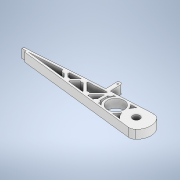
# Autodesk Inventor part: airfoil
Saved by Autodesk Inventor 2022 (Build 260153000, 153)
## iProperties
Created: 2021-03-06
Part Number: airfoil
Material: ABS Plastic
Document SubType Name: Modeling
Designer: Ferdinand Hubbard
Density: 1.06 g/cm^3
Appearance: Smooth - White
Mass: 36.0694 g
Surface Area: 132.212 cm^2
Volume: 34.0278 cm^3
Author: Ferdinand Hubbard
Autodesk Inventor part; units mm, degrees
ref_plane "YZ Plane" through (0, 0, 0) normal (1, 0, 0) x (0, 1, 0)
ref_plane "XZ Plane" through (0, 0, 0) normal (0, 1, 0) x (-1, 0, 0)
ref_plane "XY Plane" through (0, 0, 0) normal (0, 0, 1) x (1, 0, 0)
sketch "Sketch1" plane through (0, 0, 0) normal (0, 1, 0) x (-1, 0, 0)
  circle A0 centre (258.2631, 4.8308) radius 8
  spline S0 degree 4 poles (33.6209, 29.2007) (29.9061, 27.8418) (22.7215, 24.7905) (13.1918, 19.0698) (6.0464, 12.5974) (2.8487, 8.0358) (1.9781, 6.5052) knots 0 0 0 0 0 0.454638 0.631605 1 1 1 1 1
  line L0 (228.9693, 19.6719) -> (363.9561, 4.4165)
  circle A1 centre (370.8368, 3.6389) radius 4 construction
  circle A2 centre (234.1104, 5.3693) radius 11.5
  circle A3 centre (234.1104, 5.3693) radius 4
  circle A4 centre (206.3773, 7.0182) radius 8
  spline S1 degree 4 poles (6.5181, -5.2335) (7.1495, -5.5884) (14.4655, -7.5139) (22.7138, -8.7119) (35.9318, -9.9587) (48.9048, -10.4891) (62.2875, -10.9022) (78.073, -11.0572) (94.7047, -11.0677) (112.5814, -10.9208) (131.2146, -10.6471) (157.3003, -10.1275) (178.3649, -9.5608) (196.5129, -9.0389) (204.4707, -8.6918) knots 0 0 0 0 0 0.111052 0.17228 0.238392 0.309085 0.383789 0.461593 0.542487 0.625611 0.710417 0.796372 1 1 1 1 1
  line L1 (205.2712, 22.3501) -> (205.101, 22.3693)
  arc A5 (366.8619, 4.0863) -> (366.7774, 4.0976) centre (366.5513, 2.0974) ccw
  arc A6 (211.7482, -3.4099) -> (211.7084, 17.1634) centre (183.2631, 6.8218) ccw
  arc A7 (222.579, 17.5321) -> (220.8357, -4.8625) centre (234.1104, 5.3693) ccw
  arc A8 (211.7084, 17.1634) -> (205.101, 22.3693) centre (204.2043, 14.4352) ccw
  arc A9 (228.9693, 19.6719) -> (222.579, 17.5321) centre (228.0726, 11.7377) ccw
  arc A10 (204.4851, -8.6914) -> (211.7482, -3.4099) centre (204.2336, -0.7107) ccw
  arc A11 (220.8357, -4.8625) -> (227.4114, -7.9687) centre (227.1598, 0.0119) ccw
  line L2 (205.101, 22.3693) -> (228.9693, 19.6719)
  line L3 (204.4851, -8.6914) -> (227.4114, -7.9687)
  circle A12 centre (13.7692, 4.0714) radius 9.5
  circle A13 centre (13.7692, 4.0714) radius 8
  line L4 (6.5182, 10.2092) -> (6.4686, 10.2473)
  line L5 (6.5182, -2.0664) -> (6.4884, -2.0928)
  line L6 (6.3757, -3.4734) -> (8.2772, -5.8071)
  line L7 (6.2474, 11.5971) -> (7.6235, 13.6492)
  line L8 (7.6237, 9.1932) -> (7.4155, 9.361)
  line L9 (7.1111, 10.503) -> (8.7725, 14.7639)
  line L10 (7.7078, -1.1496) -> (7.6551, -1.1925)
  line L11 (7.6239, -2.4062) -> (12.536, -6.8462)
  arc A14 (6.4884, -2.0928) -> (6.3757, -3.4734) centre (7.151, -2.8417) ccw
  arc A15 (7.6551, -1.1925) -> (7.6239, -2.4062) centre (8.1604, -1.8127) ccw
  arc A16 (7.1111, 10.503) -> (7.4155, 9.361) centre (8.0428, 10.1397) ccw
  arc A17 (6.2474, 11.5971) -> (6.4686, 10.2473) centre (7.078, 11.0402) ccw
  circle A18 centre (206.3773, 7.0182) radius 9.5
  circle A19 centre (258.2631, 4.8308) radius 9.5
  line L12 (199.715, 25.2636) -> (204.715, 25.2636)
  line L13 (204.715, 21.8532) -> (204.715, 20.2636)
  line L14 (204.715, 20.2636) -> (199.715, 20.2636)
  line L15 (199.715, 20.2636) -> (199.715, 22.0923)
  line L16 (363.9561, 7.3621) -> (368.9561, 7.3621)
  line L17 (368.9561, 7.3621) -> (368.9561, 2.3621)
  line L18 (368.9561, 2.3621) -> (363.9561, 2.3621)
  line L19 (363.9561, 2.3621) -> (363.9561, 7.3621)
  line L20 (368.9561, 2.3621) -> (368.9561, 1.9548)
  arc A20 (367.0002, -0.0447) -> (368.9561, 1.9548) centre (366.9561, 1.9548) ccw
  spline S2 degree 4 poles (227.4114, -7.9687) (227.4417, -8.4597) (246.8106, -6.9409) (262.2854, -6.6719) (283.9243, -5.4893) (299.9375, -4.6081) (314.7418, -3.6091) (328.1615, -2.6489) (339.8305, -1.7709) (352.2883, -0.8813) (359.936, -0.3777) (366.0141, -0.1162) (366.8685, -0.083) knots 0 0 0 0 0 0.205018 0.312148 0.416329 0.516516 0.612219 0.702513 0.786392 0.862444 1 1 1 1 1
  spline S3 degree 4 poles (369.983, -0.0016) (369.9988, -0.0007) (370.0055, 0.0002) (370.0019, 0.001) (369.9872, 0.0018) knots 0 0 0 0 0 1 1 1 1 1
  line L21 (369.9445, -0.0037) -> (370.0215, 0.0006) construction
  arc A21 (369.9522, -0.0026) -> (370.0137, 0.0008) centre (369.9433, 0.7095) ccw construction
  line L22 (367.0002, -0.0447) -> (366.8685, -0.083)
  line L23 (34.5887, 29.5265) -> (39.5887, 29.5265)
  line L24 (39.5887, 26.3775) -> (39.5887, 24.5265)
  line L25 (39.5887, 24.5265) -> (34.5887, 24.5265)
  line L26 (34.5887, 24.5265) -> (34.5887, 28.83)
  line L27 (199.2285, 22.5921) -> (40.1023, 26.8773)
  arc A22 (16.4456, -7.6263) -> (9.2191, 15.1753) centre (13.7692, 4.0714) ccw
  spline S4 degree 3 poles (32.0186, 25.4505) (29.3529, 24.7737) (18.93, 19.4324) (14.8642, 16.0213) knots 0 0 0 0 1 1 1 1
  line L28 (39.5871, 22.0265) -> (34.5871, 22.0023)
  line L29 (32.0186, 25.4505) -> (32.0186, 21.9899)
  line L30 (32.0186, 21.9899) -> (34.5871, 22.0023)
  line L31 (39.5871, 22.0265) -> (42.0871, 22.0265)
  line L32 (42.0871, 24.1952) -> (42.0871, 22.0265)
  line L33 (197.2217, 20.4462) -> (197.2167, 17.9462)
  line L34 (197.2167, 17.9462) -> (207.215, 17.7637)
  line L35 (42.0871, 24.1952) -> (197.2217, 20.4462)
  line L36 (207.215, 17.7637) -> (207.215, 20.2046)
  line L37 (207.215, 20.2046) -> (361.1854, 2.2896)
  line L38 (361.1854, 2.2896) -> (361.2414, 2.3344)
  spline S5 degree 4 poles (21.2323, -5.3255) (22.7398, -5.5867) (33.0484, -6.8576) (45.6907, -7.3689) (62.672, -7.914) (78.3439, -8.0583) (95.0315, -8.0733) (112.8578, -7.9245) (131.5947, -7.6509) (162.8597, -7.0251) (191.7949, -6.2121) (206.033, -5.7336) (269.1523, -3.5276) knots 0 0 0 0 0 0.137245 0.208113 0.283 0.360995 0.442088 0.525416 0.610431 0.696597 1 1 1 1 1
  arc A23 (251.9278, 15.0021) -> (250.613, -4.3924) centre (258.2631, 4.8308) ccw
  arc A24 (266.732, -3.6434) -> (266.7606, 13.2763) centre (258.2631, 4.8308) ccw
  arc A25 (201.174, 17.874) -> (211.5805, -3.8375) centre (206.3773, 7.0182) ccw
  arc A26 (211.9193, 17.4124) -> (207.215, 18.7677) centre (206.3773, 7.0182) ccw
  line L39 (194.3397, 7.156) -> (207.169, 7.156) construction
  line L40 (270.2436, 4.8105) -> (270.2436, 4.851)
  line L41 (33.6209, 29.2007) -> (33.9085, 29.3057)
  arc A27 (34.5887, 28.83) -> (33.9085, 29.3057) centre (34.0822, 28.83) ccw
  arc A28 (40.1023, 26.8773) -> (39.5887, 26.3775) centre (40.0888, 26.3775) ccw
  arc A29 (199.715, 22.0923) -> (199.2285, 22.5921) centre (199.215, 22.0923) ccw
  arc A30 (205.2712, 22.3501) -> (204.715, 21.8532) centre (205.215, 21.8532) ccw
  line L42 (35.3648, 22.006) -> (77.8331, 22.006) construction
  arc A31 (34.3109, 22.0009) -> (41.3108, 22.0265) centre (37.8109, 22.006) ccw
  arc A32 (71.629, -7.979) -> (64.6326, -7.8826) centre (68.1322, -7.8309) ccw
  line L43 (69.8663, -4.7907) -> (96.8629, 22.2058)
  arc A33 (96.8152, 22.8727) -> (103.8138, 22.7432) centre (100.3141, 22.7881) ccw
  line L44 (102.1739, 22.7432) -> (145.1045, 22.7432) construction
  line L45 (128.514, -6.6859) -> (101.3594, 19.4479)
  arc A34 (135.3971, -7.6135) -> (128.3986, -7.6833) centre (131.8972, -7.5825) ccw
  line L46 (135.1957, -6.4122) -> (159.9144, 18.3065)
  arc A35 (158.2221, 21.3887) -> (165.2205, 21.2404) centre (161.7211, 21.3042) ccw
  line L47 (164.3595, 21.2404) -> (203.1162, 21.2404) construction
  line L48 (186.2459, -4.8887) -> (163.2172, 18.14)
  spline S6 degree 4 poles (270.2451, -3.4893) (274.1839, -3.2939) (289.3537, -2.5112) (304.4864, -1.5237) (322.5867, -0.2284) (334.2167, 0.6468) (346.6859, 1.537) (354.3039, 2.0388) (360.4144, 2.3022) (361.2414, 2.3344) knots 0 0 0 0 0 0.317091 0.45231 0.579943 0.698488 0.805988 1 1 1 1 1
  line L49 (270.2451, -3.4893) -> (270.2451, -3.4893)
  arc A36 (243.3991, -4.4259) -> (242.266, 16.1263) centre (234.1104, 5.3693) ccw
  arc A37 (228.6405, 17.7117) -> (225.5197, -5.0448) centre (234.1104, 5.3693) ccw
  arc A38 (192.9757, -6.1256) -> (185.9789, -6.3381) centre (189.4773, -6.2332) ccw
  line L50 (191.7646, 20.5781) -> (194.7646, 20.5781) construction
  line L51 (191.7645, 20.5781) -> (215.6, 20.5781) construction
  arc A39 (186.782, 20.6985) -> (193.7796, 20.5294) centre (190.2799, 20.5781) ccw
  arc A40 (283.9649, 11.2745) -> (290.9121, 10.4662) centre (287.4219, 10.7273) ccw
  line L52 (290.1119, 10.5593) -> (307.3754, 10.5593) construction
  line L53 (297.5649, -1.1365) -> (288.8815, 7.5462)
  arc A41 (304.509, -1.4937) -> (297.5273, -1.9501) centre (301.017, -1.7038) ccw
  line L54 (304.5089, -1.4937) -> (310.853, 4.8504)
  line L55 (304.5089, -1.4937) -> (317.6558, -1.4937) construction
  line L56 (309.0297, 7.2718) -> (302.962, 1.204)
  arc A42 (308.9851, 8.3633) -> (315.9382, 7.5543) centre (312.4616, 7.9588) ccw
  line L57 (314.7124, 7.6969) -> (325.9112, 7.6969) construction
  arc A43 (324.1284, -0.1058) -> (317.1469, -0.6132) centre (320.6378, -0.3611) ccw
  line L58 (204.4707, -8.6918) -> (204.4851, -8.6914)
  line L59 (39.6075, 22.006) -> (39.5871, 22.0265)
  line L60 (66.4718, -4.7499) -> (41.017, 20.6022)
  line L61 (98.6233, 19.7236) -> (71.5927, -7.307)
  line L62 (70.9281, -7.9716) -> (70.9277, -7.972)
  line L63 (38.7394, 18.6315) -> (64.6725, -7.3016)
  line L64 (133.7022, -7.5931) -> (133.7015, -7.5924)
  line L65 (130.4879, -4.3788) -> (103.7835, 22.3257)
  line L66 (158.2467, 20.8815) -> (133.0777, -4.2876)
  line L67 (129.7036, -7.6617) -> (129.7009, -7.6644)
  line L68 (188.7646, 17.4231) -> (188.7646, -2.8065)
  line L69 (188.7646, -6.2548) -> (188.7646, -6.2573)
  line L70 (165.1222, 20.4778) -> (188.4786, -2.8787)
  line L71 (191.7631, -6.1632) -> (191.7646, -6.1647)
  line L72 (191.7646, -6.1647) -> (191.7646, -6.1631)
  line L73 (191.7646, -3.584) -> (191.7646, 17.4086)
  line L74 (271.9866, 0.175) -> (271.9866, 9.322)
  line L75 (271.9866, -3.042) -> (287.8594, -3.042) construction
  line L76 (274.9866, 9.2013) -> (274.9867, -0.787)
  arc A44 (276.0313, -3.1918) -> (269.0412, -3.5314) centre (272.5324, -3.2823) ccw
  line L77 (285.6486, 7.7098) -> (275.8299, -2.1089)
  line L78 (274.6757, -3.263) -> (274.6567, -3.282)
  line L79 (273.7313, 0.006) -> (283.9539, 10.2547)
  arc A45 (270.1443, 12.8826) -> (277.0965, 12.0737) centre (273.6138, 12.4208) ccw
  line L80 (290.8124, 9.8587) -> (299.3172, 1.3539)
  line L81 (302.3114, -1.6402) -> (302.319, -1.6479)
  line L82 (317.3441, 0.8227) -> (313.5382, 4.6285)
  line L83 (315.7224, 6.6869) -> (319.4707, 2.9386)
  line L84 (37.8109, 18.506) -> (37.8109, -3.5678)
  line L85 (37.8109, 22.006) -> (66.7673, 22.006) construction
  line L86 (40.8109, -3.5678) -> (40.8109, 20.2032)
  arc A46 (42.7787, -7.2041) -> (35.8117, -6.804) centre (39.3109, -6.7301) ccw
  line L87 (269.1523, -3.5276) -> (270.2451, -3.4893)
  line L88 (-47.0069, 14.7639) -> (200.751, 17.2554)
  line L89 (200.751, 17.2554) -> (200.9822, -5.7446)
  line L90 (200.9822, -5.7446) -> (-46.7756, -8.2361)
  line L91 (-46.7756, -8.2361) -> (-47.0069, 14.7639)
  line L92 (82.3516, 14.4972) -> (123.3495, 14.9094)
  line L93 (123.3495, 14.9094) -> (123.5506, -5.0896)
  line L94 (123.5506, -5.0896) -> (82.5527, -5.5018)
  line L95 (82.5527, -5.5018) -> (82.3516, 14.4972)
  line L96 (201.5453, 17.8672) -> (201.5453, 20.2636)
  line L97 (275.2386, -5.5018) -> (280.2344, -5.2957)
  line L98 (280.2344, -5.2957) -> (280.7704, -18.2846)
  line L99 (278.8545, -20.3654) -> (277.8554, -20.4066)
  line L100 (275.7746, -18.4908) -> (275.2386, -5.5018)
  arc A47 (278.8545, -20.3654) -> (280.7704, -18.2846) centre (278.7721, -18.3671) ccw
  arc A48 (275.7746, -18.4908) -> (277.8554, -20.4066) centre (277.7729, -18.4083) ccw
  line L101 (277.7365, -5.3988) -> (278.2313, -17.3886) construction
  circle A49 centre (278.2313, -17.3886) radius 0.75
  point P0 (0, 0)
  point P1 (35.937, 30.0257)
  point P2 (12.8155, 18.1391)
  point P3 (3.7499, 9.1521)
  point P4 (1.2115, 4.8535)
  point P5 (0.0668, 1.0195)
  point P6 (0.0003, -0.0638)
  point P7 (0.0755, -0.9849)
  point P8 (0.2106, -1.5356)
  point P9 (0.4302, -2.0122)
  point P10 (0.7739, -2.4345)
  point P11 (1.2488, -2.8423)
  point P12 (2.1566, -3.4383)
  point P13 (3.2773, -4.0196)
  point P14 (15.3668, -7.4261)
  point P15 (24.3167, -8.7706)
  point P16 (35.0526, -9.7678)
  point P17 (47.9909, -10.4262)
  point P18 (61.6814, -10.8267)
  point P19 (77.2847, -11.0213)
  point P20 (94.162, -11.0379)
  point P21 (112.1091, -10.9014)
  point P22 (130.911, -10.6315)
  point P23 (150.3435, -10.2474)
  point P24 (170.176, -9.7646)
  point P25 (190.1737, -9.1986)
  point P26 (211.1546, -8.8311)
  point P27 (248.6815, -7.1077)
  point P28 (267.1761, -6.3211)
  point P29 (284.4085, -5.4599)
  point P30 (300.6314, -4.5262)
  point P31 (315.513, -3.5432)
  point P32 (328.9899, -2.5787)
  point P33 (340.8611, -1.7041)
  point P34 (350.9621, -0.9861)
  point P35 (359.0972, -0.4681)
  point P36 (365.0802, -0.1604)
  point P37 (368.7597, -0.0285)
  point P38 (112.1091, -11.9485)
  point P39 (1.9781, 6.5052)
  point P40 (204.3503, 22.4541)
  point P41 (204.4619, -8.7595)
  point P42 (5.7253, 10.8186)
  point P43 (5.7692, -2.729)
  point P44 (6.845, 9.8205)
  point P45 (6.9325, -1.7812)
  point P46 (46.0163, 32.9548)
  point P47 (369.983, -0.0016)
  point P48 (14.8642, 16.0213)
  point P49 (224.1134, -5.4471)
  point P50 (243.1914, -4.6981)
  point P51 (261.5022, -3.9011)
  point P52 (295.0061, -2.108)
  point P53 (309.9078, -1.1246)
  point P54 (323.3849, -0.1604)
  point P55 (335.2575, 0.7143)
  point P56 (345.3581, 1.4322)
  point P57 (353.4942, 1.9501)
  point P58 (359.4855, 2.2582)
  point P59 (8.583, -2.8113)
  point P60 (15.6728, -4.4303)
  point P61 (48.2968, -7.4304)
  point P62 (61.9872, -7.831)
  point P63 (77.5905, -8.0255)
  point P64 (94.4679, -8.0421)
  point P65 (112.4149, -7.9055)
  point P66 (131.2169, -7.636)
  point P67 (150.6492, -7.2509)
  point P68 (170.4819, -6.7695)
  point P69 (190.4797, -6.2026)
  point P70 (21.2326, -5.3256)
  point P71 (21.2326, -5.3256)
  point P72 (21.2323, -5.3255)
  point P73 (103.8131, 22.7036)
  point P74 (135.3971, -7.5616)
  point P75 (212.7436, -0.033)
  point P76 (212.6228, 14.1767)
  point P77 (211.5304, 17.6105)
  point P78 (210.0494, 19.8748)
  point P79 (205.237, 22.3528)
  point P80 (165.2201, 21.2196)
  point P81 (40.8109, 16.56)
  point P82 (77.8277, 16.0193)
  point P83 (117.8257, 16.4215)
  point P84 (200.0132, -3.2004)
  point P85 (200.0314, 17.2481)
  point P86 (16.5617, -7.5992)
  point P87 (71.8566, -7.0431)
  point P88 (9.6259, 15.3334)
  point P89 (200.9322, -0.7664)
  point P90 (200.962, -3.7334)
  point P91 (200.7767, 14.6918)
  point P92 (95.0926, 16.1929)
  point P93 (192.9535, -5.8254)
  point P94 (210.5822, -5.5532)
  point P95 (191.0213, 17.1575)
  point P96 (189.6075, 17.1433)
  point P97 (17.6852, 15.4145)
  point P98 (16.3095, -7.6017)
  point P99 (280.8528, -20.2829)
  point P100 (247.0763, 9.1258)
  point P101 (274.9867, 1.2647)
  point P102 (266.7643, -3.611)
  point P103 (275.2569, -5.9439)
  point P104 (280.2504, -5.6845)
  point P105 (246.896, 1.0386)
  point P106 (250.3677, -4.1833)
  point P107 (360.9148, 2.3211)
  dimension "d69" = 8
  dimension "d50" = 368.7594
  dimension "d57" = 16
  dimension "d70" = 23
  dimension "d71" = 8
  dimension "d73" = 16
  dimension "d80" = 19
  dimension "d81" = 16
  dimension "d82" = 1
  dimension "d83" = 1
  dimension "d84" = 1
  dimension "d85" = 1
  dimension "d86" = 1
  dimension "d87" = 0.8
  dimension "d88" = 1
  dimension "d90" = 19
  dimension "d94" = 5
  dimension "d95" = 5
  dimension "d105" = 5
  dimension "d106" = 5
  dimension "d108" = 2
  dimension "d109" = 19
  dimension "d114" = 5
  dimension "d115" = 5
  dimension "d116" = 24
  dimension "d117" = 2.5
  dimension "d118" = 2.5
  dimension "d123" = 2.5
  dimension "d124" = 2.5
  dimension "d125" = 10
  dimension "d135" = 0.5
  dimension "d186" = 45
  dimension "d197" = 90
  dimension "d203" = 90
  dimension "d209" = 40
  dimension "d212" = 41
  dimension "d213" = 20
  dimension "d214" = 23
  dimension "d215" = 5
  dimension "d216" = 15
  dimension "d217" = 2
  dimension "d218" = 12
  dimension "d219" = 1.5
  constraints: 200 end point, 136 point on circle, 49 centre point, 32 tangent, 31 point on line, 15 horizontal, 13 parallel, 11 coincident, 7 perpendicular, 6 equal radius, 3 collinear, 3 midpoint, 3 vertical, 133 other
  measures "d50" distance of point (368.76, -0.028) point (0, -0.064)
  measures "d57" diameter of A0
  measures "d70" diameter of A2
  measures "d71" diameter of A3
  measures "d73" diameter of A4
  measures "d80" diameter of A12
  measures "d81" diameter of A13
  measures "d82" distance of L4.start point (5.725, 10.819)
  measures "d83" distance of L5.start point (5.769, -2.729)
  measures "d84" distance of L8.start point (6.845, 9.821)
  measures "d85" distance of L10.start point (6.933, -1.781)
  measures "d86" radius of A14
  measures "d87" radius of A15
  measures "d88" radius of A16
  measures "d90" diameter of A19
  measures "d94" distance of L13.end L14.end
  measures "d95" distance of L12.end L13.end
  measures "d105" distance of L17.end L18.end
  measures "d106" distance of L16.end L17.end
  measures "d108" radius of A20
  measures "d109" diameter of A18
  measures "d114" distance of L24.end L25.end
  measures "d115" distance of L23.end L24.end
  measures "d116" diameter of A22
  measures "d117" distance of L24.end L28.start
  measures "d118" distance of L28.start L31.end
  measures "d123" distance of L14.end L33.start
  measures "d124" distance of L33.start L33.end
  measures "d125" distance of L33.end L34.end
  measures "d135" radius of A29
  measures "d186" angle of L55 L54
  measures "d197" angle of L75 L74
  measures "d203" angle of L84 L85
  measures "d209" distance of point (77.828, 16.019) point (117.826, 16.421)
  measures "d212" distance of L92.start L92.end
  measures "d213" distance of L92.end L93.end
  measures "d214" vertical distance of L90.end L88.start
  measures "d215" distance of L97.start L97.end
  measures "d216" distance of L97.end point (280.853, -20.283)
  measures "d217" radius of A47
  measures "d218" distance of L101.start L101.end
  measures "d219" diameter of A49
extrude "Extrusion6" add sketch "Sketch1" along normal blind 10 contours A11 S5 A2 A19 L87 S6 L37 A9 L0 L19 L18 L20 A20 L22 S2 L98 L97 L100 | A11 A7 A9 L37 A37 S5 | L100 L97 L98 S2 | S2 L98 A47 L99 A48 L100 | A37 L37 A36 A23 S5 A2 | S5 A2 | A2 S5 | L37 A19 S5 A23 A36 | A36 A23 | L37 A24 S5 A19 | L37 A45 | A44 S6 L87 S5 | A45 L76 L79 A44 L74 | L37 A40 | L79 L76 A44 | A40 L77 A44 L76 L79 | L37 A42 | L80 A41 L53 A40 | A42 L54 A41 L56 | A41 S6 | L83 A43 L82 A42 | S6 A43
body "Solid6"
